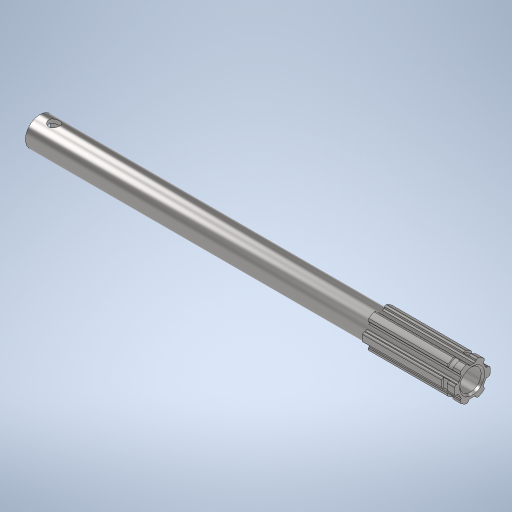
# Autodesk Inventor part: Shaft
Saved by Autodesk Inventor 2023.2 (Build 272271000, 271)
## iProperties
Created: 2024-01-10
Part Number: Shaft
Material: Stainless Steel
Document SubType Name: Modeling
Designer: Nathan Cai
Density: 8 g/cm^3
Appearance: Semi-Polished
Mass: 23.8639 g
Surface Area: 55.7927 cm^2
Volume: 2.98298 cm^3
Author: Nathan Cai
Autodesk Inventor part; units mm, degrees
ref_plane "YZ Plane" through (0, 0, 0) normal (1, 0, 0) x (0, 1, 0)
ref_plane "XZ Plane" through (0, 0, 0) normal (0, 1, 0) x (-1, 0, 0)
ref_plane "XY Plane" through (0, 0, 0) normal (0, 0, 1) x (1, 0, 0)
sketch "Sketch1" plane through (0, 0, 0) normal (1, 0, 0) x (0, 1, 0)
  circle A0 centre (0, 0) radius 4
  circle A1 centre (0, 0) radius 3
  dimension "d0" = 8
  dimension "d1" = 6
  constraints: 2 centre point, 2 coincident
  measures "d0" diameter of A0
  measures "d1" diameter of A1
extrude "Extrusion1" add sketch "Sketch1" along normal blind 120
sketch "Sketch2" plane through (120, 0, 0) normal (1, 0, 0) x (0, 0, -1)
  line L0 (-0.0955, 0) -> (4, 0) construction
  circle A0 centre (0, 0) radius 4 projected
  line L1 (4.8412, 1.25) -> (0, 1.25)
  line L2 (0, 1.25) -> (0, -1.25) construction
  line L3 (0, -1.25) -> (4.8412, -1.25)
  line L4 (4.8412, -1.25) -> (4.8412, 1.25) construction
  line L5 (4.8412, 1.25) -> (0, -1.25) construction
  line L6 (0, 1.25) -> (4.8412, -1.25) construction
  circle A1 centre (0, 0) radius 5
  line L7 (-0.0477, -0.0827) -> (2, 3.4641) construction
  line L8 (1.3381, 4.8176) -> (-1.0825, 0.625)
  line L9 (-1.0825, 0.625) -> (1.0825, -0.625) construction
  line L10 (1.0825, -0.625) -> (3.5031, 3.5676)
  line L11 (3.5031, 3.5676) -> (1.3381, 4.8176) construction
  line L12 (1.3381, 4.8176) -> (1.0825, -0.625) construction
  line L13 (-1.0825, 0.625) -> (3.5031, 3.5676) construction
  line L14 (0.0477, -0.0827) -> (-2, 3.4641) construction
  line L15 (-3.5031, 3.5676) -> (-1.0825, -0.625)
  line L16 (-1.0825, -0.625) -> (1.0825, 0.625) construction
  line L17 (1.0825, 0.625) -> (-1.3381, 4.8176)
  line L18 (-1.3381, 4.8176) -> (-3.5031, 3.5676) construction
  line L19 (-3.5031, 3.5676) -> (1.0825, 0.625) construction
  line L20 (-1.0825, -0.625) -> (-1.3381, 4.8176) construction
  line L21 (0.0955, 0) -> (-4, 0) construction
  line L22 (-4.8412, -1.25) -> (0, -1.25)
  line L23 (0, -1.25) -> (0, 1.25) construction
  line L24 (0, 1.25) -> (-4.8412, 1.25)
  line L25 (-4.8412, 1.25) -> (-4.8412, -1.25) construction
  line L26 (-4.8412, -1.25) -> (0, 1.25) construction
  line L27 (0, -1.25) -> (-4.8412, 1.25) construction
  line L28 (0.0477, 0.0827) -> (-2, -3.4641) construction
  line L29 (-1.3381, -4.8176) -> (1.0825, -0.625)
  line L30 (1.0825, -0.625) -> (-1.0825, 0.625) construction
  line L31 (-1.0825, 0.625) -> (-3.5031, -3.5676)
  line L32 (-3.5031, -3.5676) -> (-1.3381, -4.8176) construction
  line L33 (-1.3381, -4.8176) -> (-1.0825, 0.625) construction
  line L34 (1.0825, -0.625) -> (-3.5031, -3.5676) construction
  line L35 (-0.0477, 0.0827) -> (2, -3.4641) construction
  line L36 (3.5031, -3.5676) -> (1.0825, 0.625)
  line L37 (1.0825, 0.625) -> (-1.0825, -0.625) construction
  line L38 (-1.0825, -0.625) -> (1.3381, -4.8176)
  line L39 (1.3381, -4.8176) -> (3.5031, -3.5676) construction
  line L40 (3.5031, -3.5676) -> (-1.0825, -0.625) construction
  line L41 (1.0825, 0.625) -> (1.3381, -4.8176) construction
  point P0 (2.4206, 0)
  point P1 (1.2103, 2.0963)
  point P2 (-1.2103, 2.0963)
  point P3 (-2.4206, 0)
  point P4 (-1.2103, -2.0963)
  point P5 (1.2103, -2.0963)
  point P6 (-2.9824, -2.6656)
  point P7 (-3.5031, -3.5676)
  point P8 (-1.3381, -4.8176)
  point P9 (-0.8173, -3.9156)
  point P10 (0.8173, -3.9156)
  point P11 (1.3381, -4.8176)
  point P12 (3.5031, -3.5676)
  point P13 (2.9824, -2.6656)
  point P14 (4.8412, 1.25)
  point P15 (3.7997, 1.25)
  point P16 (3.7997, -1.25)
  point P17 (2.9824, 2.6656)
  point P18 (3.5031, 3.5676)
  point P19 (1.3381, 4.8176)
  point P20 (0.8173, 3.9156)
  point P21 (-3.7997, 1.25)
  point P22 (-4.8412, -1.25)
  point P23 (-3.7997, -1.25)
  point P24 (-0.8173, 3.9156)
  point P25 (-1.3381, 4.8176)
  point P26 (-3.5031, 3.5676)
  point P27 (-2.9824, 2.6656)
  dimension "d23" = 10
  dimension "d21" = 2.5
  dimension "d26" = 360
  constraints: 84 end point, 18 midpoint, 12 point on line, 8 coincident, 3 parallel, 1 horizontal, 1 perpendicular, 106 other
  measures "d21" distance of L2.end L1.end
extrude "Extrusion2" add sketch "Sketch2" against normal blind 25.5 contours A0 L1 A1 L3 | A0 L8 A1 L10 | L36 A1 L38 A0 | A0 L15 A1 L17 | L29 A1 L31 A0 | A0 L22 A1 L24
fillet "Fillet1" radius 0.5 24 edges at (107.25, 4.8176, 1.3381) (107.25, 3.5676, 3.5031) (107.25, 4.8176, -1.3381) (107.25, 3.5676, -3.5031) (107.25, 1.25, -4.8412) (107.25, -1.25, -4.8412) (107.25, -3.5676, -3.5031) (107.25, -4.8176, -1.3381) (107.25, -4.8176, 1.3381) (107.25, -3.5676, 3.5031) (107.25, -1.25, 4.8412) (107.25, 1.25, 4.8412) (107.25, 3.9156, -0.8173) (107.25, 3.9156, 0.8173) (107.25, 2.6656, -2.9824) (107.25, 1.25, -3.7997) (107.25, -1.25, -3.7997) (107.25, -2.6656, -2.9824) (107.25, -3.9156, -0.8173) (107.25, -3.9156, 0.8173) (107.25, -2.6656, 2.9824) (107.25, -1.25, 3.7997) (107.25, 1.25, 3.7997) (107.25, 2.6656, 2.9824)
sketch "Sketch3" plane through (0, 0, 0) normal (0, 1, 0) x (-1, 0, 0)
  line L0 (0, 0) -> (-120, 0) construction
  line L1 (-120, -3) -> (-120, 3) projected
  circle A0 centre (-4, 0) radius 1.5
  circle A1 centre (-4, 0) radius 4
  line L2 (0, 4) -> (-94.5, 4) projected
  line L3 (0, 4) -> (0, -4) projected
  line L4 (-8, -4) -> (0, -4)
  line L5 (0, -4) -> (0, 4)
  line L6 (0, 4) -> (-8, 4)
  line L7 (-8, 4) -> (-8, -4)
  line L8 (-8, -4) -> (0, 4) construction
  line L9 (0, -4) -> (-8, 4) construction
  point P0 (-4, 4)
  point P1 (-4, -4)
  point P2 (0, -4)
  dimension "d10" = 3
  constraints: 14 end point, 3 midpoint, 2 centre point, 2 parallel, 2 tangent, 1 coincident, 1 horizontal, 1 perpendicular, 1 point on line
  measures "d10" diameter of A0
extrude "Extrusion3" cut sketch "Sketch3" along normal through all both and the other way through all contours A0
ref_plane "Work Plane1" through (118, 0, 0) normal (1, 0, 0) x (0, 0, -1)
sketch "Sketch4" plane through (118, 0, 0) normal (1, 0, 0) x (0, 0, -1)
  arc A0 (3.6851, -1.5556) -> (3.6851, 1.5556) centre (0, 0) ccw projected
  circle A1 centre (0, 0) radius 6
  circle A2 centre (0, 0) radius 10
  circle A3 centre (0, 0) radius 4.5
  arc A4 (0.4954, 3.9692) -> (-0.4954, 3.9692) centre (0, 0) ccw projected
  point P0 (5.7956, 1.5529)
  point P1 (5.7956, -1.5529)
  point P2 (6, 0)
  point P3 (3.7997, -1.25)
  point P4 (3.7997, 1.25)
  dimension "d14" = 20
  dimension "d29" = 9
  constraints: 2 centre point, 2 coincident, 3 other
  measures "d14" diameter of A2
  measures "d29" diameter of A3
extrude "Extrusion4" cut sketch "Sketch4" against normal blind 1.5 contours A1 | A2
chamfer "Chamfer1" distance 0.5 angle 45 1 edges at (120, -3, 0)
body "Solid1"
